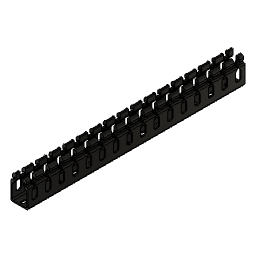
Parametric Wire Ducts v5 (Autodesk Fusion 360 design; units mm, degrees)
Autodesk Fusion 360 part; units mm, degrees
note: some values were not read from the file. Set by a fixed rule: which sketch regions a step uses.
sketch "Cross section" plane through (0, 0, 0) normal (0, 1, 0) x (1, 0, 0)
  line L0 (0, 0) -> (25, 0) construction
  line L1 (25, 0) -> (25, -40) construction
  line L2 (25, -40) -> (0, -40) construction
  line L3 (0, -40) -> (0, 0) construction
  line L4 (0, -40) -> (25, -40)
  line L5 (0, 0) -> (25, 0)
  line L6 (4.3598, -28.2) -> (5.7, -29.5402)
  line L7 (0, -40) -> (0, -24.6887) construction
  line L8 (0, -24.6887) -> (5.1, -29.7887) construction
  line L9 (1.6, -30.4) -> (1.6, -38.4)
  line L10 (1.6, -38.4) -> (23.4, -38.4)
  line L11 (1.6, -38.4) -> (1.6, -1.6) construction
  line L12 (1.6, -1.6) -> (23.4, -1.6)
  line L13 (23.4, -1.6) -> (23.4, -38.4) construction
  line L14 (5.7, -29.5402) -> (5.7, -33.5)
  line L15 (1.6, -23.1775) -> (7.3, -28.8775)
  line L16 (7.3, -28.8775) -> (7.3, -37.8)
  line L17 (0, -28.8) -> (4.1113, -28.8)
  line L18 (0, -28.8) -> (0, -40)
  line L19 (0, -28.2) -> (0, 0)
  line L20 (1.6, -23.1775) -> (1.6, -1.6)
  line L21 (2.2, -31) -> (2.2, -33.8)
  line L22 (7.3, -37.8) -> (6.2, -37.8)
  arc A0 (2.2, -33.8) -> (6.2, -37.8) centre (6.2, -33.8) ccw
  line L23 (2.2, -31) -> (3.2, -31)
  line L24 (3.2, -31) -> (5.7, -33.5)
  line L25 (5.1, -29.7887) -> (5.1, -32.0515)
  line L26 (1.6, -30.4) -> (3.4485, -30.4)
  line L27 (3.4485, -30.4) -> (5.1, -32.0515)
  line L28 (1.6, -30.4) -> (3.4485, -30.4)
  line L29 (4.1113, -28.8) -> (5.1, -29.7887)
  line L30 (12.5, -40) -> (12.5, 0) construction
  line L31 (4.3598, -28.2) -> (0, -28.2)
  line L32 (17.7, -28.8775) -> (17.7, -37.8)
  line L33 (23.4, -23.1775) -> (17.7, -28.8775)
  line L34 (23.4, -23.1775) -> (23.4, -1.6)
  line L35 (19.3, -29.5402) -> (19.3, -33.5)
  line L36 (19.9, -29.7887) -> (19.9, -32.0515)
  line L37 (21.5515, -30.4) -> (19.9, -32.0515)
  line L38 (21.8, -31) -> (19.3, -33.5)
  line L39 (22.8, -31) -> (21.8, -31)
  arc A1 (18.8, -37.8) -> (22.8, -33.8) centre (18.8, -33.8) ccw
  line L40 (22.8, -31) -> (22.8, -33.8)
  line L41 (17.7, -37.8) -> (18.8, -37.8)
  line L42 (20.6402, -28.2) -> (19.3, -29.5402)
  line L43 (25, -28.8) -> (20.8887, -28.8)
  line L44 (20.6402, -28.2) -> (25, -28.2)
  line L45 (25, -28.2) -> (25, 0)
  line L46 (20.8887, -28.8) -> (19.9, -29.7887)
  line L47 (23.4, -30.4) -> (21.5515, -30.4)
  line L48 (23.4, -30.4) -> (23.4, -38.4)
  line L49 (25, -28.8) -> (25, -40)
  dimension "d1" = 25
  dimension "d4" = 40
  dimension "d7" = 1.6
  dimension "d9" = 1.6
  dimension "d13" = 1.6
  dimension "d14" = 1.6
  dimension "d18" = 0.6
  dimension "d23" = 4
  dimension "d24" = 1
  dimension "d25" = 45
  dimension "d26" = 0.6
  dimension "d27" = 0.6
  dimension "d28" = 0.6
  dimension "d29" = 1.6
  dimension "d31" = 0.6
  dimension "d32" = 0.6
  dimension "d33" = 3.5
  dimension "d34" = 1.6
  dimension "d35" = 1.6
  dimension "d36" = 8
  dimension "d37" = 1.6
  dimension "d38" = 0.6
  constraint horizontal L0
  constraint vertical L1
  constraint horizontal L2
  constraint vertical L3
  constraint coincident L0.start L3.end
  constraint coincident L3 L19.start
  constraint coincident L3 L7.end
  constraint vertical L9
  constraint perpendicular L9 L10
  constraint perpendicular L10 L11
  constraint perpendicular L11 L12
  constraint vertical L13
  constraint vertical L14
  constraint coincident L14 L24.end
  constraint coincident L11 L15.start
  constraint parallel L6 L15
  constraint parallel L6 L8
  constraint coincident L7 L17.start
  constraint coincident L8 L17.end
  constraint perpendicular L11 L17
  constraint perpendicular L21 L22
  constraint horizontal L22
  constraint tangent L22 A0
  constraint tangent L21 A0
  constraint perpendicular L21 L23
  constraint vertical L25
  constraint perpendicular L11 L26
  constraint parallel L24 L27
  constraint coincident L9 L26.start
  constraint coincident L27 L26.end
  constraint perpendicular L9 L28
  constraint midpoint L4 L30.start
  constraint midpoint L5 L30.end
  constraint coincident L7 L19.start
  constraint horizontal L31
  constraint coincident L19.start L31.end
  constraint symmetric L19.start L30 L44.end
  constraint symmetric L6.end L30 L35.start
  constraint symmetric L8.end L30 L36.start
  constraint symmetric L9.end L30 L10.end
  constraint symmetric L11.end L30 L12.end
  constraint symmetric L21.start L30 L39.start
  constraint symmetric L14.end L30 L35.end
  constraint symmetric L15.start L30 L33.start
  constraint symmetric L15.end L30 L32.start
  constraint symmetric L16.end L30 L32.end
  constraint symmetric L17.start L30 L43.start
  constraint symmetric L17.end L30 L43.end
  constraint symmetric L0.start L30 L0.end
  constraint symmetric L22.end L30 A1.start
  constraint symmetric L21.end L30 A1.end
  constraint symmetric A0 L30 A1
  constraint symmetric L23.end L30 L38.start
  constraint symmetric L25.end L30 L36.end
  constraint symmetric L26.end L30 L37.start
  constraint symmetric L9.start L30 L47.start
  constraint symmetric L30 L6.start L42.start
  constraint symmetric L30 L19.start L44.end
  measures "d1" distance of L0.start L0.end
  measures "d4" distance of L0.start L2.end
  measures "d7" distance of L4 L10
  measures "d9" distance of L5 L12
  measures "d13" distance of L14 L16
  measures "d14" distance of L6 L15
  measures "d18" distance of L6 L8
  measures "d23" radius of A0
  measures "d24" distance of L21.start L23.end
  measures "d25" angle of L14 L24
  measures "d26" distance of L14 L25
  measures "d27" distance of L24 L27
  measures "d28" distance of L23 L26
  measures "d29" distance of L8 L27
  measures "d31" distance of L10 L22
  measures "d32" distance of L9 L21
  measures "d33" distance of L14 L21
  measures "d34" distance of L11 L19
  measures "d35" distance of L17 L26
  measures "d36" distance of L10 L26
  measures "d37" distance of L1 L13
  measures "d38" distance of L17 L31
extrude "Extrude1" add sketch "Cross section" along normal blind 320 contours L4 L9 L10 L17 L18 L25 L26 L27 L28 L29 L36 L37 L43 L46 L47 L48 L49 makes body 1
extrude "Extrude2" add sketch "Cross section" along normal blind 320 separate body contours L5 L6 L12 L14 L15 L16 L19 L20 L21 L22 A0 L23 L24 L31 L32 L33 L34 L35 L38 L39 A1 L40 L41 L42 L44 L45 makes body 2
chamfer "Chamfer1" distance 1 angle 45 2 edges at (25, 160, 0) (0, 160, 0) on bodies 2
fillet "Fillet10" radius 2 2 edges at (1.6, 160, 1.6) (23.4, 160, 1.6) on bodies 2
fillet "Fillet9" radius 2 2 edges at (25, 160, 1) (0, 160, 1) on bodies 2
fillet "Fillet1" radius 3 4 edges at (1.6, 160, 23.1775) (7.3, 160, 28.8775) (17.7, 160, 28.8775) (23.4, 160, 23.1775) on bodies 2
fillet "Fillet2" radius 2 2 edges at (0, 160, 28.2) (25, 160, 28.2) on bodies 2
chamfer "Chamfer2" distance 1 angle 45 2 edges at (25, 160, 28.8) (0, 160, 28.8) on bodies 1
fillet "Fillet3" radius 2 4 edges at (19.9, 160, 29.7887) (5.1, 160, 29.7887) (0, 160, 29.8) (25, 160, 29.8) on bodies 1
fillet "Fillet5" radius 0.4 4 edges at (5.1, 160, 32.0515) (19.9, 160, 32.0515) (19.3, 160, 33.5) (5.7, 160, 33.5) on bodies 1 2
fillet "Fillet6" [suppressed]
fillet "Fillet7" radius 1 2 edges at (17.7, 160, 37.8) (7.3, 160, 37.8) on bodies 2
fillet "Fillet8" radius 1 2 edges at (0, 160, 40) (25, 160, 40) on bodies 1
sketch "Side cutouts" plane through (25, 0, 0) normal (1, 0, 0) x (0, 1, 0)
  line L0 (320, 26.2) -> (0, 26.2)
  line L1 (0, 26.2) -> (0, 1.8284)
  line L2 (320, 1.8284) -> (320, 26.2)
  line L3 (6, 38.8) -> (14, 38.8) construction
  line L4 (14, 38.8) -> (14, 31.7426) construction
  line L5 (14, 9) -> (6, 9) construction
  line L6 (6, 31.7426) -> (6, 38.8) construction
  line L7 (0, 0) -> (320, 0) construction
  line L8 (0, 1.8284) -> (320, 1.8284)
  line L9 (10, 38.8) -> (10, 9) construction
  line L10 (9.2803, 25.9803) -> (6.8787, 23.5787)
  line L11 (9.5, 26.5107) -> (9.5, 26.6893)
  line L12 (9.2803, 27.2197) -> (6.8787, 29.6213)
  line L13 (6, 21.4574) -> (6, 11)
  line L14 (14, 11) -> (6, 11) construction
  arc A0 (6.25, 10.6928) -> (13.75, 10.6928) centre (10, 14) ccw
  line L15 (6, 22.7) -> (14, 22.7) construction
  line L16 (14, 21.4574) -> (14, 11.3542)
  line L17 (10.5, 26.5107) -> (10.5, 26.6893)
  line L18 (10.5, 27) -> (9.5, 27) construction
  line L19 (10.7197, 25.9803) -> (13.1213, 23.5787)
  line L20 (6, 30.5) -> (14, 30.5) construction
  line L21 (10.7197, 27.2197) -> (13.1213, 29.6213)
  line L22 (6, 30.5) -> (6, 38.8)
  line L23 (6, 38.8) -> (14, 38.8)
  line L24 (14, 38.8) -> (14, 30.5)
  line L25 (0, 37.8) -> (320, 37.8)
  arc A1 (6.8787, 23.5787) -> (6, 21.4574) centre (9, 21.4574) ccw
  arc A2 (14, 21.4574) -> (13.1213, 23.5787) centre (11, 21.4574) ccw
  arc A3 (6, 11.3542) -> (6.25, 10.6928) centre (7, 11.3542) ccw
  arc A4 (13.75, 10.6928) -> (14, 11.3542) centre (13, 11.3542) ccw
  arc A5 (6, 31.7426) -> (6.8787, 29.6213) centre (9, 31.7426) ccw
  arc A6 (13.1213, 29.6213) -> (14, 31.7426) centre (11, 31.7426) ccw
  arc A7 (9.2803, 25.9803) -> (9.5, 26.5107) centre (8.75, 26.5107) ccw
  arc A8 (9.5, 26.6893) -> (9.2803, 27.2197) centre (8.75, 26.6893) ccw
  arc A9 (10.7197, 27.2197) -> (10.5, 26.6893) centre (11.25, 26.6893) ccw
  arc A10 (10.5, 26.5107) -> (10.7197, 25.9803) centre (11.25, 26.5107) ccw
  point P0 (9.5, 26.2)
  dimension "d63" = 8
  dimension "d65" = 6
  dimension "d66" = 9
  dimension "d72" = 2
  dimension "d73" = 1
  dimension "d74" = 0.8
  dimension "d75" = 45
  dimension "d76" = 1
  dimension "d77" = 45
  dimension "d91" = 3
  dimension "d92" = 1
  dimension "d93" = 3
  dimension "d94" = 0.75
  dimension "d95" = 0.75
  dimension "d96" = 0.3542
  constraint horizontal L3
  constraint vertical L4
  constraint horizontal L5
  constraint vertical L6
  constraint midpoint L3 L9.start
  constraint midpoint L5 L9.end
  constraint coincident L0 P0
  constraint coincident L6 L15.start
  constraint perpendicular L0 L11
  constraint coincident L6 L20.start
  constraint coincident L6 L13.end
  constraint coincident L4 L14.start
  constraint horizontal L14
  constraint coincident L9.end A0
  constraint coincident L4 L15.end
  constraint perpendicular L4 L15
  constraint perpendicular L0 L17
  constraint perpendicular L11 L18
  constraint symmetric L9 L11 L17
  constraint coincident L4 L20.end
  constraint perpendicular L4 L20
  constraint perpendicular L3 L22
  constraint coincident L15.start L10
  constraint coincident L15.start L13
  constraint tangent L10 A1
  constraint tangent L13 A1
  constraint coincident L15.end L19
  constraint coincident L15.end L16
  constraint tangent L19 A2
  constraint tangent L16 A2
  constraint equal A1 A2
  constraint tangent A0 A3
  constraint tangent L6 A3
  constraint coincident L14.start L16
  constraint coincident L14.start A0
  constraint tangent A0 A4
  constraint tangent L16 A4
  constraint equal A3 A4
  constraint coincident L20.start L12
  constraint coincident L6 A3.start
  constraint tangent L12 A5
  constraint tangent L6 A5
  constraint coincident L20.end L21
  constraint coincident L5.start L4
  constraint tangent L21 A6
  constraint tangent L4 A6
  constraint equal A5 A6
  constraint coincident P0 L10
  constraint coincident P0 L11
  constraint tangent L10 A7
  constraint tangent L11 A7
  constraint coincident L18.end L11
  constraint coincident L18.end L12
  constraint tangent L11 A8
  constraint tangent L12 A8
  constraint equal A7 A8
  constraint coincident L18.start L17
  constraint coincident L18.start L21
  constraint tangent L17 A9
  constraint tangent L21 A9
  constraint equal A7 A9
  constraint tangent L19 A10
  constraint tangent L17 A10
  constraint horizontal A7.centre A10.centre
  measures "d63" distance of L4 L6
  measures "d65" distance of L1 L6
  measures "d66" distance of L5 L7
  measures "d72" distance of L5 L14
  measures "d73" distance of L11 L17
  measures "d74" distance of P0 L18.end
  measures "d75" angle of L10 L15
  measures "d76" distance of L23 L25
  measures "d77" angle of L12 L20
  measures "d91" radius of A1
  measures "d92" radius of A3
  measures "d93" radius of A5
  measures "d94" radius of A7
  measures "d95" radius of A10
  measures "d96" distance of L14 A3.centre
extrude "Extrude3" cut sketch "Side cutouts" against normal up to surface (25 mm away) contours L0 L10 L13 A0 L16 L19 A1 A2 A3 A4 A7 A10 | L0 L11 L12 L17 L21 L22 L24 L25 A5 A6 A7 A8 A9 A10 | L22 L23 L24 L25 bodies 2
pattern_linear "R-Pattern1" count 16 spacing 20 along (0, 1, 0) of "Extrude3"
sketch "Screw holes" plane through (0, 0, 0) normal (0, 0, -1) x (1, 0, 0)
  line L0 (1, 0) -> (1, -320)
  line L1 (1, -320) -> (24, -320)
  line L2 (24, -320) -> (24, 0)
  line L3 (24, 0) -> (1, 0)
  line L4 (12.5, 0) -> (12.5, -320) construction
  line L5 (10.25, -4.75) -> (10.25, -8.25)
  arc A0 (10.25, -8.25) -> (14.75, -8.25) centre (12.5, -8.25) ccw
  line L6 (14.75, -8.25) -> (14.75, -4.75)
  arc A1 (14.75, -4.75) -> (10.25, -4.75) centre (12.5, -4.75) ccw
  line L7 (12.5, -4.75) -> (12.5, -8.25) construction
  point P0 (12.5, -2.5)
  dimension "d97" = 4.5
  dimension "d98" = 3.5
  dimension "d99" = 2.5
  constraint midpoint L3 L4.start
  constraint midpoint L1 L4.end
  constraint tangent L5 A0
  constraint tangent A0 L6
  constraint parallel L5 L6
  constraint tangent L6 A1
  constraint tangent L5 A1
  constraint coincident L4 A0.centre
  constraint parallel L4 L7
  constraint midpoint A1 P0
  measures "d97" diameter of A0
  measures "d98" distance of A1.centre A0.centre
  measures "d99" distance of L4.start P0
extrude "Extrude4" cut sketch "Screw holes" against normal up to surface (1.6 mm away) contours L5 A0 L6 A1 bodies 2
pattern_linear "R-Pattern2" count 13 spacing 25 along (0, 1, 0) of "Extrude4"
hidden bodies 1
equation "d1 = ductWidth"
equation "ductWidth = 25 mm"
equation "ductHeight = 40 mm"
equation "d4 = ductHeight"
equation "thickness = 1.6 mm"
equation "d7 = thickness"
equation "d9 = thickness"
equation "d13 = thickness"
equation "d14 = thickness"
equation "d18 = partsGapTolerance"
equation "partsGapTolerance = 0.6 mm"
equation "interiorSlopeAngle = 45 deg"
equation "d26 = partsGapTolerance"
equation "d27 = partsGapTolerance"
equation "d28 = partsGapTolerance"
equation "d29 = thickness"
equation "d31 = partsGapTolerance"
equation "d32 = partsGapTolerance"
equation "d34 = thickness"
equation "d35 = thickness"
equation "d37 = thickness"
equation "d38 = partsGapTolerance"
equation "ductLength = 320 mm"
equation "d40 = ductLength"
equation "d42 = ductLength"
equation "cutoutWidth = 8 mm"
equation "d63 = cutoutWidth"
equation "cutoutSpacing = 12 mm"
equation "d65 = cutoutSpacing / 2"
equation "cutouts = ductLength / ( cutoutSpacing + cutoutWidth )"
equation "d87 = cutouts"
equation "d89 = cutoutSpacing + cutoutWidth"
equation "d93 = d91"
equation "d95 = d94"
equation "d97 = screwSlotWidth"
equation "d98 = screwSlotLengthCenters"
equation "d102 = screwSlots"
equation "d104 = screwSlotSpacing"
equation "screwSlotWidth = 4.5 mm"
equation "screwSlotLengthCenters = screwSlotWidth - 1 mm"
equation "screwSlotSpacing = 25 mm"
equation "screwSlots = ceil(ductLength / screwSlotSpacing)"
named bodies: "Top", "Base"
